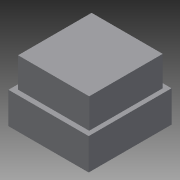
# Autodesk Inventor part: hobbyking150acaresc
Saved by Autodesk Inventor 2014 (Build 180170000, 170)
## iProperties
Created: 2014-05-21
Part Number: hobbyking150acaresc
Material: Generic
Document SubType Name: Modeling
Designer: brent
Density: 1 g/cm^3
Appearance: Default
Author: brent
Autodesk Inventor part; units mm, degrees
ref_plane "YZ Plane" through (0, 0, 0) normal (1, 0, 0) x (0, 1, 0)
ref_plane "XZ Plane" through (0, 0, 0) normal (0, 1, 0) x (-1, 0, 0)
ref_plane "XY Plane" through (0, 0, 0) normal (0, 0, 1) x (1, 0, 0)
sketch "Sketch1" plane through (0, 0, 0) normal (0, 1, 0) x (-1, 0, 0)
  line L0 (0, 0) -> (54.56, 0)
  line L1 (54.56, 0) -> (54.56, -56.34)
  line L2 (54.56, -56.34) -> (0, -56.34)
  line L3 (0, -56.34) -> (0, 0)
  dimension "d0" = 56.34
  dimension "d1" = 54.56
  constraints: 8 end point, 2 parallel, 1 horizontal, 1 perpendicular
  measures "d0" distance of L2.end L0.start
  measures "d1" distance between parallel lines of L3 L1
extrude "Extrusion1" add sketch "Sketch1" along normal blind 21.4
sketch "Sketch2" plane through (0, 21.4, 0) normal (0, 1, 0) x (1, 0, 0)
  line L0 (0, 0) -> (0, 56.34) projected
  line L1 (0, 56.34) -> (-54.56, 56.34) projected
  line L2 (-51.36, 53.34) -> (-3, 53.34)
  line L3 (-3, 53.34) -> (-3, 3.34)
  line L4 (-3, 3.34) -> (-51.36, 3.34)
  line L5 (-51.36, 3.34) -> (-51.36, 53.34)
  dimension "d4" = 48.36
  dimension "d5" = 50
  dimension "d6" = 3
  dimension "d7" = 3
  constraints: 8 end point, 2 parallel, 1 horizontal, 1 perpendicular
  measures "d4" distance between parallel lines of L5 L3
  measures "d5" distance between parallel lines of L4 L2
  measures "d6" distance between parallel lines of L1 L2
  measures "d7" distance between parallel lines of L0 L3
extrude "Extrusion2" add sketch "Sketch2" along normal blind 20.25
body "Solid1"
